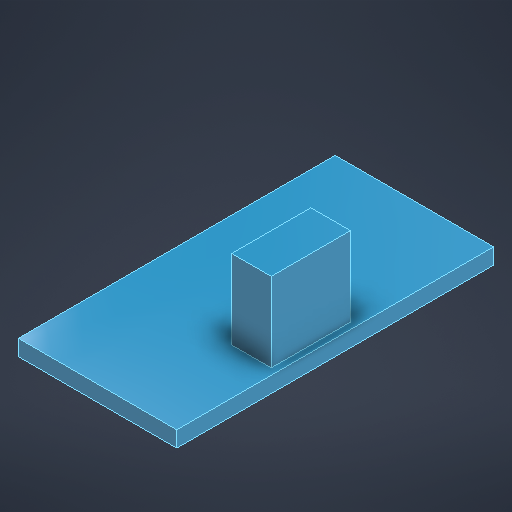
# Autodesk Inventor part: boost-converter
Saved by Autodesk Inventor 2025.2 (Build 292293000, 293)
## iProperties
Created: 2025-12-22
Part Number: boost-converter
Material: ABS Plastic
Document SubType Name: Modeling
Designer: sam
Density: 1.06 g/cm^3
Appearance: Sky Blue Dark
Author: sam
Autodesk Inventor part; units mm, degrees
ref_plane "YZ Plane" through (0, 0, 0) normal (1, 0, 0) x (0, 1, 0)
ref_plane "XZ Plane" through (0, 0, 0) normal (0, 1, 0) x (-1, 0, 0)
ref_plane "XY Plane" through (0, 0, 0) normal (0, 0, 1) x (1, 0, 0)
sketch "Sketch1" plane through (0, 0, 0) normal (0, 1, 0) x (-1, 0, 0)
  line L0 (-8, -16) -> (8, -16)
  line L1 (8, -16) -> (8, 16)
  line L2 (8, 16) -> (-8, 16)
  line L3 (-8, 16) -> (-8, -16)
  line L4 (-8, -16) -> (8, 16) construction
  line L5 (8, -16) -> (-8, 16) construction
  point P0 (0, 0)
  dimension "d0" = 16
  dimension "d1" = 32
  constraints: 12 end point, 2 midpoint, 2 parallel, 1 horizontal, 1 perpendicular
  measures "d0" distance of L2.end L1.end
  measures "d1" distance of L1.end L0.end
extrude "Extrusion1" add sketch "Sketch1" along normal blind 1.6
sketch "Sketch2" plane through (0, 1.6, 0) normal (0, 1, 0) x (1, 0, 0)
  line L0 (3.3525, 2.1899) -> (7.3525, 2.1899)
  line L1 (7.3525, 2.1899) -> (7.3525, -5.8101)
  line L2 (7.3525, -5.8101) -> (3.3525, -5.8101)
  line L3 (3.3525, -5.8101) -> (3.3525, 2.1899)
  point P0 (0, 0)
  dimension "d4" = 4
  dimension "d5" = 8
  constraints: 8 end point, 2 parallel, 1 horizontal, 1 perpendicular
  measures "d4" distance of L1.end L2.end
  measures "d5" distance of L0.end L1.end
extrude "Extrusion2" add sketch "Sketch2" along normal blind 8
body "Solid1"
